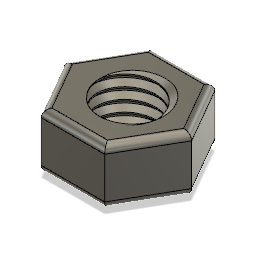
22part (Autodesk Fusion 360 design; units mm, degrees)
Autodesk Fusion 360 part; units mm, degrees
sketch "Sketch1" plane through (0, 0, 0) normal (0, 1, 0) x (1, 0, 0)
  circle A0 centre (0, 0) radius 2.5
  line L0 (-2.3094, 4) -> (-4.6188, 0)
  line L1 (-4.6188, 0) -> (-2.3094, -4)
  line L2 (-2.3094, -4) -> (2.3094, -4)
  line L3 (2.3094, -4) -> (4.6188, 0)
  line L4 (4.6188, 0) -> (2.3094, 4)
  line L5 (2.3094, 4) -> (-2.3094, 4)
  dimension "d1" = 5
  dimension "d2" = 4
  constraint coincident A0.centre origin
  constraint horizontal L5
  measures "d1" diameter of A0
  measures "d2" distance of A0.centre L5
extrude "Extrude1" add sketch "Sketch1" along normal blind 4
fillet "Fillet1" radius 0.5 12 edges at (0, 0, -4) (-3.4641, 0, -2) (-3.4641, 0, 2) (0, 0, 4) (3.4641, 0, 2) (3.4641, 0, -2) (0, 4, 4) (3.4641, 4, 2) (3.4641, 4, -2) (0, 4, -4) (-3.4641, 4, -2) (-3.4641, 4, 2)
thread "Thread1" "ISO Metric profile 5.0 M5x0.8 6H" major diameter 5.12 minor diameter 4.234 pitch 0.8 angle 60 modelled right hand crest width 0.1 on face at (2.4969, 2.6667, 0.1246) crest through (2.117, -0.45, 0)
